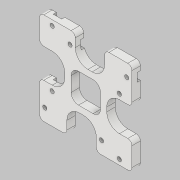
# Autodesk Inventor part: BaseBottom
Saved by Autodesk Inventor 2019.2 (Build 232265000, 265)
## iProperties
Created: 2019-01-12
Part Number: BaseBottom
Material: ABS-Kunststoff
Document SubType Name: Modeling
Designer: Lion
Density: 1.06 g/cm^3
Appearance: Weiß
Mass: 4.77958 g
Surface Area: 42.0374 cm^2
Volume: 4.50904 cm^3
Author: Lion
## iProperties of the stored document BaseBottom_3D-Druck.ipt
Created: 2019-04-11
Part Number: BaseBottom_3D-Druck
Material: Generisch
Document SubType Name: Modeling
Designer: Lion
Density: 1 g/cm^3
Appearance: Vorgabe
Author: Lion
Autodesk Inventor part; units mm, degrees
note: some values were not read from the file. Chosen so that the rebuilt part matches the saved one: sketch regions of "Base".
ref_plane "YZ Plane" through (0, 0, 0) normal (1, 0, 0) x (0, 1, 0)
ref_plane "XZ Plane" through (0, 0, 0) normal (0, 1, 0) x (-1, 0, 0)
ref_plane "XY Plane" through (0, 0, 0) normal (0, 0, 1) x (1, 0, 0)
sketch "Skizze2" plane through (0, 0, 0) normal (0, 0, 1) x (1, 0, 0)
  line L0 (-16, -6) -> (16, -6)
  line L1 (16, -6) -> (16, 6)
  line L2 (16, 6) -> (-16, 6)
  line L3 (-16, 6) -> (-16, -6)
  line L4 (-16, -6) -> (16, 6) construction
  line L5 (16, -6) -> (-16, 6) construction
  line L6 (-11, 6) -> (3, 6)
  line L7 (3, 6) -> (3, -6)
  line L8 (3, -6) -> (-11, -6)
  line L9 (-11, -6) -> (-11, 6)
  circle A0 centre (-13.5, 0) radius 1
  line L10 (-11, -6) -> (-16, 6) construction
  line L11 (-16, -6) -> (-11, 6) construction
  line L12 (0, 6) -> (0, -6) construction
  circle A1 centre (13.5, 0) radius 1
  line L13 (-16, -26) -> (-16, 6)
  line L14 (-16, 6) -> (-28, 6)
  line L15 (-28, 6) -> (-28, -26)
  line L16 (-28, -26) -> (-16, -26)
  line L17 (-16, -26) -> (-28, 6) construction
  line L18 (-16, 6) -> (-28, -26) construction
  line L19 (-28, -21) -> (-28, -7)
  line L20 (-28, -7) -> (-16, -7)
  line L21 (-16, -7) -> (-16, -21)
  line L22 (-16, -21) -> (-28, -21)
  circle A2 centre (-22, -23.5) radius 1
  line L23 (-16, -21) -> (-28, -26) construction
  line L24 (-16, -26) -> (-28, -21) construction
  line L25 (-28, -10) -> (-16, -10) construction
  circle A3 centre (-22, 3.5) radius 1
  line L26 (-1, -26) -> (4, -38) construction
  line L27 (-15, -38) -> (-15, -26)
  line L28 (-12, -38) -> (-12, -26) construction
  line L29 (4, -26) -> (-28, -26)
  line L30 (-28, -38) -> (4, -38)
  line L31 (4, -26) -> (-28, -38) construction
  line L32 (-28, -26) -> (4, -38) construction
  line L33 (-1, -26) -> (-1, -38)
  line L34 (-15, -26) -> (-1, -26)
  line L35 (4, -26) -> (-1, -38) construction
  line L36 (4, -38) -> (4, -26)
  circle A4 centre (1.5, -32) radius 1
  line L37 (-1, -38) -> (-15, -38)
  circle A5 centre (-25.5, -32) radius 1
  line L38 (-28, -26) -> (-28, -38)
  line L39 (4, -11) -> (16, -6) construction
  line L40 (16, -25) -> (4, -25)
  line L41 (16, -22) -> (4, -22) construction
  line L42 (4, -6) -> (4, -38)
  line L43 (16, -38) -> (16, -6)
  line L44 (4, -6) -> (16, -38) construction
  line L45 (4, -38) -> (16, -6) construction
  line L46 (4, -11) -> (16, -11)
  line L47 (4, -25) -> (4, -11)
  line L48 (4, -6) -> (16, -11) construction
  line L49 (16, -6) -> (4, -6)
  circle A6 centre (10, -8.5) radius 1
  line L50 (16, -11) -> (16, -25)
  circle A7 centre (10, -35.5) radius 1
  line L51 (4, -38) -> (16, -38)
  line L52 (-16, -26) -> (4, -6) construction
  line L53 (4, -26) -> (-16, -6) construction
  line L54 (1, -23) -> (-13, -23)
  line L55 (-13, -23) -> (-13, -9)
  line L56 (-13, -9) -> (1, -9)
  line L57 (1, -9) -> (1, -23)
  line L58 (1, -23) -> (-13, -9) construction
  line L59 (-13, -23) -> (1, -9) construction
  line L60 (4, -25) -> (16, -25)
  line L61 (16, -25) -> (16, -38)
  line L62 (16, -38) -> (4, -38)
  line L63 (4, -38) -> (4, -25)
  point P0 (0, 0)
  point P1 (-13.5, 0)
  point P2 (-22, -10)
  point P3 (-12, -32)
  point P4 (10, -22)
  point P5 (-6, -16)
  dimension "d9" = 32
  dimension "d10" = 12
  dimension "d11" = 5
  dimension "d12" = 14
  dimension "d13" = 2
  dimension "d14" = 32
  dimension "d15" = 12
  dimension "d16" = 5
  dimension "d17" = 14
  dimension "d18" = 2
  dimension "d19" = 32
  dimension "d20" = 12
  dimension "d21" = 5
  dimension "d22" = 14
  dimension "d23" = 2
  dimension "d24" = 32
  dimension "d25" = 12
  dimension "d26" = 5
  dimension "d27" = 14
  dimension "d28" = 2
  dimension "d29" = 3
  constraints: 128 end point, 20 parallel, 20 point on line, 16 midpoint, 14 perpendicular, 8 centre point, 4 coincident, 4 horizontal, 4 symmetric about line, 2 collinear, 4 other
  measures "d9" distance of L2.end L1.end
  measures "d10" distance of L1.end L0.end
  measures "d11" distance between parallel lines of L3 L9
  measures "d12" distance between parallel lines of L7 L9
  measures "d13" diameter of A0
  measures "d14" distance of L23.end L15.start
  measures "d15" distance of L2.end L15.start
  measures "d16" distance between parallel lines of L16 L22
  measures "d17" distance between parallel lines of L20 L22
  measures "d18" diameter of A2
  measures "d19" distance of L32.end L38.end
  measures "d20" distance of L23.end L38.end
  measures "d21" distance between parallel lines of L36 L33
  measures "d22" distance between parallel lines of L27 L33
  measures "d23" diameter of A4
  measures "d24" distance of L45.end L51.end
  measures "d25" distance of L32.end L51.end
  measures "d26" distance between parallel lines of L49 L46
  measures "d27" distance between parallel lines of L40 L46
  measures "d28" diameter of A6
  measures "d29" distance between parallel lines of L8 L56
extrude "Base" add sketch "Skizze2" along normal blind 4 contours L3 L2 L9 L0 | L13 L20 L15 L14 L3 | L0 L42 L29 L13 | L7 L2 L1 L0 | L13 L16 L15 L22 | L0 L43 L46 L42 | L29 L27 L30 L38 L16 | L40 L43 L51 L36 L42 | L29 L36 L30 L33
fillet "Rundung1" radius 3.5 4 edges at (1, -9, 2) (1, -23, 2) (-13, -23, 2) (-13, -9, 2)
fillet "Rundung2" radius 6 8 edges at (-1, -26, 2) (-15, -26, 2) (-16, -21, 2) (-16, -7, 2) (-11, -6, 2) (3, -6, 2) (4, -11, 2) (4, -25, 2)
sketch "Skizze4" plane through (0, 0, 0) normal (0, 0, -1) x (-1, 0, 0)
  circle A0 centre (-13.5, 0) radius 1 projected
  circle A1 centre (22, 3.5) radius 1 projected
  circle A2 centre (25.5, -32) radius 1 projected
  circle A3 centre (-10, -35.5) radius 1 projected
  circle A4 centre (22, 3.5) radius 2
  circle A5 centre (25.5, -32) radius 2
  circle A6 centre (-10, -35.5) radius 2
  circle A7 centre (-13.5, 0) radius 2
  line L0 (-16, 6) -> (-16, -11) construction
  line L1 (-16, -38) -> (1, -38) construction
  line L2 (28, -38) -> (28, -21) construction
  line L3 (28, 6) -> (11, 6) construction
  line L4 (20, 3.5) -> (20, 6)
  line L5 (24, 3.5) -> (24, 6)
  line L6 (20, 6) -> (24, 6)
  line L7 (25.5, -30) -> (28, -30)
  line L8 (28, -34) -> (25.5, -34)
  line L9 (28, -30) -> (28, -34)
  line L10 (-12, -35.5) -> (-12, -38)
  line L11 (-8, -35.5) -> (-8, -38)
  line L12 (1, -38) -> (-16, -38) projected
  line L13 (-8, -38) -> (-12, -38)
  line L14 (-13.5, 2) -> (-16, 2)
  line L15 (-16, 2) -> (-16, -2)
  line L16 (-16, -2) -> (-13.5, -2)
  circle A8 centre (-10, -8.5) radius 2
  circle A9 centre (-10, -8.5) radius 1 projected
  circle A10 centre (-1.5, -32) radius 1 projected
  circle A11 centre (22, -23.5) radius 1 projected
  circle A12 centre (13.5, 0) radius 1 projected
  circle A13 centre (13.5, 0) radius 2
  circle A14 centre (22, -23.5) radius 2
  circle A15 centre (-1.5, -32) radius 2
  line L17 (-1.5, -30) -> (1.3431, -30)
  line L18 (1.3431, -30) -> (1.3431, -34)
  line L19 (1.3431, -34) -> (-1.5, -34)
  arc A16 (7, -26) -> (1, -32) centre (7, -32) ccw projected
  line L20 (20, -23.5) -> (20, -20.6569)
  line L21 (20, -20.6569) -> (24, -20.6569)
  line L22 (24, -20.6569) -> (24, -23.5)
  arc A17 (16, -15) -> (22, -21) centre (22, -15) ccw projected
  line L23 (-8, -8.5) -> (-8, -11.3431)
  line L24 (-8, -11.3431) -> (-12, -11.3431)
  line L25 (-12, -11.3431) -> (-12, -8.5)
  arc A18 (-4, -17) -> (-10, -11) centre (-10, -17) ccw projected
  line L26 (13.5, -2) -> (10.6569, -2)
  arc A19 (5, -6) -> (11, 0) centre (5, 0) ccw projected
  line L27 (10.6569, -2) -> (10.6569, 2)
  line L28 (10.6569, 2) -> (13.5, 2)
  point P0 (0, 0)
  dimension "screwhead_d" = 4
  dimension "d45" = 4
  dimension "d46" = 4
  dimension "d47" = 4
  dimension "d50" = 4
  dimension "d52" = 4
  dimension "d54" = 4
  dimension "d56" = 4
  constraints: 48 end point, 20 point on circle, 16 tangent, 14 perpendicular, 8 centre point, 8 coincident, 8 point on line, 3 collinear, 3 horizontal, 3 vertical
  measures "screwhead_d" diameter of A4
  measures "d45" diameter of A5
  measures "d46" diameter of A6
  measures "d47" diameter of A7
  measures "d50" diameter of A8
  measures "d52" diameter of A13
  measures "d54" diameter of A14
  measures "d56" diameter of A15
extrude "Extrusion3" cut sketch "Skizze4" against normal blind 1.5 contours A0 | A1 | A2 | A4 | A4 L4 L6 L5 | A5 | A5 L7 L9 L8 | A6 | L11 L12 L10 A6 | A7 | A7 L16 L15 L14 | A8 | L23 L24 L25 A8 | A9 | A10 | A11 | A12 | A13 | A13 L26 L27 L28 | A14 | A14 L20 L21 L22 | A15 | A15 L17 L18 L19
fillet "Rundung3" radius 2 12 edges at (-28, -38, 2) (-28, 6, 2) (16, 6, 2) (16, -38, 2) (3, 6, 2) (-11, 6, 2) (16, -11, 2) (16, -25, 2) (-1, -38, 2) (-15, -38, 2) (-28, -7, 2) (-28, -21, 2)
fillet "Rundung4" [suppressed]
